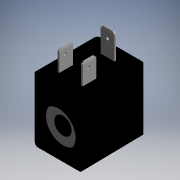
# Autodesk Inventor part: 389924 MSFG-24-42-50/60---(P)
Saved by Autodesk Inventor 2021 (Build 250183000, 183)
## iProperties
Part Number: 389924 MSFG-24-42-50/60---(P)
Material: Genérico
Catalog Web Link: www.cadenas.de
Description: MSFG-p-Solenoid coil
Vendor: FESTO
Document SubType Name: Modeling
Designer: partserver
Manufacturer: FESTO
Mass: 16.7159 g
Surface Area: 53.6023 cm^2
Volume: 16.7159 cm^3
Density: 1 g/cm^3
Appearance: PSOLRGB-0-0-0
Category: PARTsolutions
Company: FESTO
PSOL_IDENT_0: {$CADENAS_DATA\23d-libs\festo\parts\m\msfg\parts\msfg_part.prj},198 {VTYP=3D},{NB=389924 MSFG-24-42-
PSOL_IDENT_1: 50/60---(P)},{LINA=389924 MSFG-24-42-50/60---(P)},{NN=MSFG-p},{DATE=07.12.2017 08:58:26},{GEOMDATE=0
PSOL_IDENT_2: 7.12.2017 08:58:00},{VERSION=},{LINEID=30},{WBVAR=},{WBNUMERIC=}  {NB=389924 MSFG-24-42-50/60---(P)}
PSOL_IDENT_3: ,{LINA=389924 MSFG-24-42-50/60---(P)},{KT=DUMMY},{TNR=389924},{TYP=MSFG-24-42-50/60},{VERS=1}
NB: 389924 MSFG-24-42-50/60---(P)
NN: MSFG-p
NT: Solenoid coil
NBSYN: $TNR. $TYP.---(P)
LINA: 389924 MSFG-24-42-50/60---(P)
CATALOG: Festo
TNR: 389924
TYP: MSFG-24-42-50/60
VERS: 1
SUPPLIER: FESTO
ARTICLENO: 389924 MSFG-24-42-50/60---(P)
BOMINFO: 389924 MSFG-24-42-50/60---(P)
CREATOR: CADENAS GmbH
Title: 389924 MSFG-24-42-50/60---(P)
Author: Cadenas PARTsolutions
Comments: Solenoid coil
Autodesk Inventor part; units mm, degrees
sketch "Sketch_2" plane through (0, 0, 0) normal (1, 0, 0) x (0, 1, 0)
  line L0 (0, 29.5) -> (0, 0)
  line L1 (0, 0) -> (29, 0)
  line L2 (29, 0) -> (29, 27.5198)
  arc A0 (29, 27.5198) -> (27.5262, 29.0195) centre (27.5, 27.5198) ccw
  line L3 (27.5262, 29.0195) -> (0, 29.5)
  constraints: 8 end point, 2 point on circle, 1 centre point
extrude "Extrusion1" add sketch "Sketch_2" along normal mid plane 22
sketch "Sketch_3" plane through (0, 0, 0) normal (0, 0.9998, -0.0175) x (1, 0, 0)
  line L0 (-11, -28) -> (-11, -38)
  line L1 (-11, -38) -> (11, -38)
  line L2 (11, -38) -> (11, -28)
  arc A0 (9.5, -29.5) -> (11, -28) centre (9.5, -28) ccw
  line L3 (9.5, -29.5) -> (-9.5, -29.5)
  arc A1 (-11, -28) -> (-9.5, -29.5) centre (-9.5, -28) ccw
  constraints: 8 end point, 4 point on circle, 2 centre point
extrude "Extrusion2" cut sketch "Sketch_3" along normal mid plane 60
sketch "Sketch_4" plane through (0, 0, 0) normal (0, 0, 1) x (1, 0, 0)
  arc A0 (-9.5, 29) -> (-11, 27.5) centre (-9.5, 27.5) ccw
  line L0 (-9.5, 29) -> (9.5, 29)
  arc A1 (11, 27.5) -> (9.5, 29) centre (9.5, 27.5) ccw
  line L1 (11, 27.5) -> (11, 37.5)
  line L2 (11, 37.5) -> (-11, 37.5)
  line L3 (-11, 37.5) -> (-11, 27.5)
  constraints: 8 end point, 4 point on circle, 2 centre point
extrude "Extrusion3" cut sketch "Sketch_4" along normal blind 29.5
sketch "Sketch_5" plane through (0, 0, 0) normal (1, 0, 0) x (0, 1, 0)
  line L0 (0, 17) -> (29, 17)
  line L1 (29, 17) -> (29, 9.15)
  line L2 (29, 9.15) -> (27.5, 9.15)
  line L3 (27.5, 9.15) -> (27.5, 13)
  line L4 (27.5, 13) -> (2, 13)
  line L5 (2, 13) -> (2, 9.15)
  line L6 (2, 9.15) -> (0, 9.15)
  line L7 (0, 9.15) -> (0, 17)
  line L8 (0, 17) -> (29, 17)
  constraints: 18 end point
revolve "Revolution1" cut sketch "Sketch_5" angle 360 about axis through (0, 0, 17) along (0, -1, 0)
sketch "Sketch_16" plane through (0, 0, 0) normal (0, 0, 1) x (1, 0, 0)
  arc A0 (-7.85, 3.5) -> (-6.35, 2) centre (-6.35, 3.5) ccw
  line L0 (-6.35, 2) -> (6.35, 2)
  arc A1 (6.35, 2) -> (7.85, 3.5) centre (6.35, 3.5) ccw
  line L1 (7.85, 3.5) -> (7.85, 24.1)
  arc A2 (7.85, 24.1) -> (6.35, 25.6) centre (6.35, 24.1) ccw
  line L2 (6.35, 25.6) -> (-6.35, 25.6)
  arc A3 (-6.35, 25.6) -> (-7.85, 24.1) centre (-6.35, 24.1) ccw
  line L3 (-7.85, 24.1) -> (-7.85, 3.5)
  constraints: 8 end point, 8 point on circle, 4 centre point
extrude "Extrusion4" cut sketch "Sketch_16" along normal blind 0.1
sketch "Sketch6" plane through (0, 0, 0.1) normal (0, 0, -1) x (-1, 0, 0)
  point P0 (0, 14.5)
hole "Hole1" at (0, 14.5, 0.1) direction (0, 0, 1) diameter 2.459 depth 6 tip angle 120 countersink diameter 3 countersink angle 90 thread size "M3x0.5" class "6H" standard "ISO Metric profile"
sketch "Sketch_18" plane through (0, 0, 0) normal (1, 0, 0) x (0, 1, 0)
  line L0 (23.4, 0.1) -> (22.6, 0.1)
  line L1 (22.6, 0.1) -> (22.6, -10.5)
  line L2 (22.6, -10.5) -> (22.8, -11.5)
  line L3 (22.8, -11.5) -> (23.2, -11.5)
  line L4 (23.2, -11.5) -> (23.4, -10.5)
  line L5 (23.4, -10.5) -> (23.4, 0.1)
  constraints: 12 end point
extrude "Extrusion5" add sketch "Sketch_18" along normal mid plane 6.3
sketch "Sketch_7" plane through (0, 8.5, 0) normal (0, 1, 0) x (1, 0, 0)
  line L0 (5, 8.5) -> (5, -0.1)
  line L1 (5, -0.1) -> (5.8, -0.1)
  line L2 (5.8, -0.1) -> (5.8, 8.5)
  line L3 (5.8, 8.5) -> (5.6, 9.5)
  line L4 (5.6, 9.5) -> (5.2, 9.5)
  line L5 (5.2, 9.5) -> (5, 8.5)
  constraints: 12 end point
extrude "Extrusion6" add sketch "Sketch_7" along normal mid plane 6.3
sketch "Sketch_8" plane through (0, 8.5, 0) normal (0, 1, 0) x (1, 0, 0)
  line L0 (-5.8, 8.5) -> (-5.8, -0.1)
  line L1 (-5.8, -0.1) -> (-5, -0.1)
  line L2 (-5, -0.1) -> (-5, 8.5)
  line L3 (-5, 8.5) -> (-5.2, 9.5)
  line L4 (-5.2, 9.5) -> (-5.6, 9.5)
  line L5 (-5.6, 9.5) -> (-5.8, 8.5)
  constraints: 12 end point
extrude "Extrusion7" add sketch "Sketch_8" along normal mid plane 6.3
sketch "Sketch_10" plane through (0, 0, 0) normal (0, 1, 0) x (-1, 0, 0)
  circle A0 centre (0, -7.5) radius 0.65
  constraints: 1 centre point
extrude "Extrusion8" cut sketch "Sketch_10" along normal blind 29
sketch "Sketch_11" plane through (0, 0, 0) normal (1, 0, 0) x (0, 1, 0)
  circle A0 centre (8.15, -6.1) radius 0.65
  constraints: 1 centre point
extrude "Extrusion9" cut sketch "Sketch_11" along normal mid plane 22
sketch "Sketch_12" plane through (0, 0, 0) normal (0, 1, 0) x (-1, 0, 0)
  line L0 (3.15, -10.5) -> (1.7358, -11.9142)
  line L1 (1.7358, -11.9142) -> (-1.7358, -11.9142)
  line L2 (-1.7358, -11.9142) -> (-3.15, -10.5)
  line L3 (-3.15, -10.5) -> (-3.15, -12.5)
  line L4 (-3.15, -12.5) -> (3.15, -12.5)
  line L5 (3.15, -12.5) -> (3.15, -10.5)
  constraints: 12 end point
extrude "Extrusion10" cut sketch "Sketch_12" along normal blind 29
sketch "Sketch_13" plane through (0, 0, 0) normal (1, 0, 0) x (0, 1, 0)
  line L0 (11.65, -8.5) -> (10.2358, -9.9142)
  line L1 (10.2358, -9.9142) -> (6.7642, -9.9142)
  line L2 (6.7642, -9.9142) -> (5.35, -8.5)
  line L3 (5.35, -8.5) -> (5.35, -10.5)
  line L4 (5.35, -10.5) -> (11.65, -10.5)
  line L5 (11.65, -10.5) -> (11.65, -8.5)
  constraints: 12 end point
extrude "Extrusion11" cut sketch "Sketch_13" along normal mid plane 22
ref_plane "2DUMMY_XY" through (0, 14.5, 0) normal (0, 0, -1) x (1, 0, 0)
ref_plane "2DUMMY_YZ" through (0, 14.5, 0) normal (1, 0, 0) x (0, -1, 0)
ref_plane "2DUMMY_ZX" through (0, 14.5, 0) normal (0, -1, 0) x (0, 0, -1)
ref_plane "ANBAU_Stecker_XY" through (0, 14.5, 0) normal (0, 0, 1) x (1, 0, 0)
ref_plane "ANBAU_Stecker_YZ" through (0, 14.5, 0) normal (1, 0, 0) x (0, 1, 0)
ref_plane "ANBAU_Stecker_ZX" through (0, 14.5, 0) normal (0, 1, 0) x (0, 0, 1)
ref_plane "IP1_XY" through (0, 27.5, 17) normal (0, -1, 0) x (1, 0, 0)
ref_plane "IP1_YZ" through (0, 27.5, 17) normal (1, 0, 0) x (0, 0, 1)
ref_plane "IP1_ZX" through (0, 27.5, 17) normal (0, 0, 1) x (0, -1, 0)
body "Solid1"
